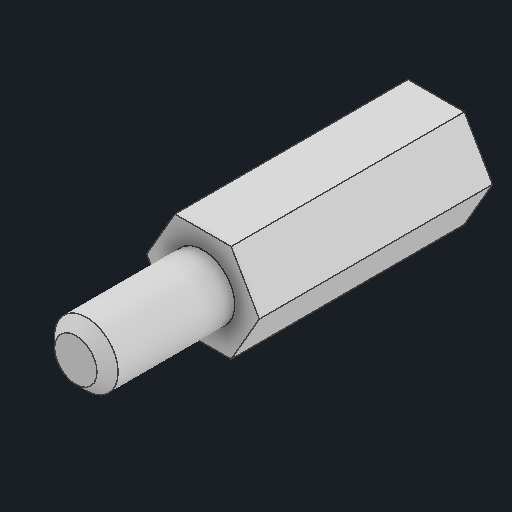
# Autodesk Inventor part: UXCell-M3x11-MaleFemaleHexStandoff
Saved by Autodesk Inventor 2025.2 (Build 292293000, 293)
## iProperties
Created: 2025-09-22
Part Number: UXCell-M3x11-MaleFemaleHexStandoff
Material: Generic
Document SubType Name: Modeling
Designer: valer
Density: 1 g/cm^3
Appearance: Default
Author: valer
Autodesk Inventor part; units mm, degrees
ref_plane "YZ Plane" through (0, 0, 0) normal (1, 0, 0) x (0, 1, 0)
ref_plane "XZ Plane" through (0, 0, 0) normal (0, 1, 0) x (-1, 0, 0)
ref_plane "XY Plane" through (0, 0, 0) normal (0, 0, 1) x (1, 0, 0)
sketch "Base" plane through (0, 0, 0) normal (0, 0, 1) x (1, 0, 0)
  line L0 (1.3279, 2.3) -> (2.6558, 0)
  line L1 (2.6558, 0) -> (1.3279, -2.3)
  line L2 (1.3279, -2.3) -> (-1.3279, -2.3)
  line L3 (-1.3279, -2.3) -> (-2.6558, 0)
  line L4 (-2.6558, 0) -> (-1.3279, 2.3)
  line L5 (-1.3279, 2.3) -> (1.3279, 2.3)
  line L6 (-3.7181, 0) -> (3.7181, 0) construction
  line L7 (0, -3.22) -> (0, 3.22) construction
  point P0 (0, 0)
  point P1 (0, 0)
  dimension "d0" = 4.6
  constraints: 12 end point, 1 coincident, 1 perpendicular, 13 other
  measures "d0" distance between parallel lines of L2 L5
extrude "BaseFeature" add sketch "Base" along normal blind 11
sketch "Sketch2" plane through (0, 0, 11) normal (0, 0, 1) x (1, 0, 0)
  circle A0 centre (0, 0) radius 1.5
  dimension "d3" = 3
  constraints: 1 centre point, 1 coincident
  measures "d3" diameter of A0
extrude "Extrusion2" add sketch "Sketch2" along normal blind 6
chamfer "Chamfer1" distance 0.5 angle 45 1 edges at (-1.5, 0, 17)
sketch "Sketch3" plane through (0, 0, 0) normal (0, 0, -1) x (-1, 0, 0)
  circle A0 centre (0, 0) radius 1.5
  dimension "d9" = 3
  constraints: 1 centre point, 1 coincident
  measures "d9" diameter of A0
extrude "Extrusion3" cut sketch "Sketch3" against normal blind 6
body "Solid1"
